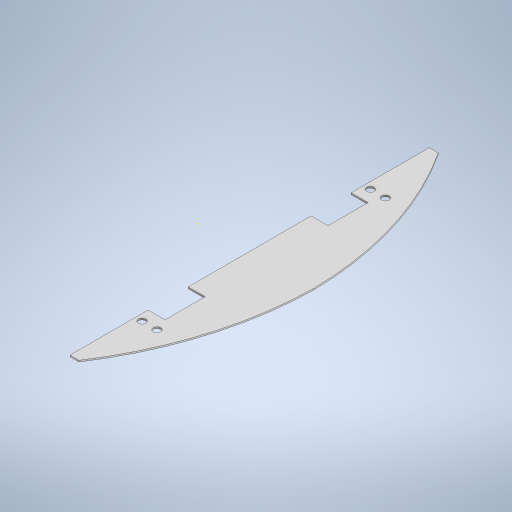
# Autodesk Inventor part: sensores1
Saved by Autodesk Inventor 2023 (Build 270158000, 158)
## iProperties
Created: 2023-08-09
Part Number: sensores1
Material: Genérico
Document SubType Name: Modeling
Designer: azeve
Density: 1 g/cm^3
Appearance: Padrão
Author: azeve
Autodesk Inventor part; units mm, degrees
ref_plane "YZ Plane" through (0, 0, 0) normal (1, 0, 0) x (0, 1, 0)
ref_plane "XZ Plane" through (0, 0, 0) normal (0, 1, 0) x (-1, 0, 0)
ref_plane "XY Plane" through (0, 0, 0) normal (0, 0, 1) x (1, 0, 0)
sketch "Esboço1" plane through (0, 0, 0) normal (0, 1, 0) x (-1, 0, 0)
  line L0 (-30.1128, 0) -> (-45.5357, 0)
  line L1 (-34.1868, -120) -> (-40.1868, -120)
  arc A0 (-76.9634, 0) -> (-40.1868, -120) centre (147.3829, 3.1204) ccw
  line L2 (-34.1868, -67.7964) -> (-45.5357, -67.7964)
  line L3 (-45.5357, -67.7964) -> (-45.5357, -41.1109)
  line L4 (-45.5357, -41.1109) -> (-34.1868, -41.1109)
  line L5 (-34.1868, 0) -> (-34.1868, -41.1109)
  line L6 (-34.1868, -67.7964) -> (-34.1868, -120)
  circle A1 centre (-38.629, -76.2964) radius 2.5
  circle A2 centre (-38.629, -76.2964) radius 2.5
  circle A3 centre (-48.643, -76.2964) radius 2.5086
  line L7 (-34.1868, 120) -> (-40.1868, 120)
  arc A4 (-40.1868, 120) -> (-76.9634, 0) centre (147.3829, -3.1204) ccw
  line L8 (-34.1868, 67.7964) -> (-45.5357, 67.7964)
  line L9 (-45.5357, 67.7964) -> (-45.5357, 41.1109)
  line L10 (-45.5357, 41.1109) -> (-34.1868, 41.1109)
  line L11 (-34.1868, 0) -> (-34.1868, 41.1109)
  line L12 (-34.1868, 67.7964) -> (-34.1868, 120)
  circle A5 centre (-38.629, 76.2964) radius 2.5
  circle A6 centre (-48.643, 76.2964) radius 2.5086
  point P0 (0, 0)
  point P1 (0, 0)
  dimension "d0" = 120
  dimension "d1" = 6
  constraints: 26 end point, 10 symmetric about line, 7 centre point, 5 perpendicular, 4 point on circle, 2 coincident, 2 vertical, 1 horizontal, 1 point on line, 3 other
  measures "d0" distance of L5.start L1.start
  measures "d1" distance of L1.start L1.end
extrude "Extrusão1" add sketch "Esboço1" along normal blind 1
sketch "Esboço2" plane through (0, 0, 0) normal (0, 1, 0) x (-1, 0, 0)
  point P0 (0, 0)
sketch "Esboço3" plane through (0, 0, 0) normal (0, -1, 0) x (1, 0, 0)
  line L0 (45.5357, 41.1109) -> (45.5357, 67.7964) projected
  line L1 (45.5357, 41.1109) -> (45.5357, 52.7605)
  point P0 (0, 0)
  constraints: 2 end point, 1 point on line, 1 vertical
